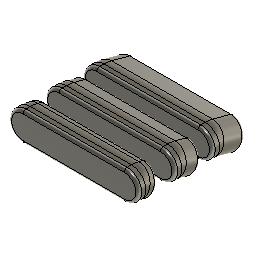
ID.3 Qi charger phone offset (Autodesk Fusion 360 design; units mm, degrees)
part number: 2026-03-30-21-57-16-208
Autodesk Fusion 360 part; units mm, degrees
sketch "Sketch2" plane through (0, 0, 0) normal (0, 1, 0) x (1, 0, 0)
  line L0 (10, 0) -> (80, 0)
  line L1 (80, -20) -> (10, -20)
  arc A0 (0, -10) -> (10, -20) centre (10, -10) ccw
  arc A1 (10, 0) -> (0, -10) centre (10, -10) ccw
  arc A2 (90, -10) -> (80, 0) centre (80, -10) ccw
  arc A3 (80, -20) -> (90, -10) centre (80, -10) ccw
  point P0 (90, 0)
  point P1 (0, -20)
  dimension "d3" = 90
  dimension "d4" = 20
  dimension "d5" = 10
  constraint horizontal L0
  constraint horizontal L1
  constraint coincident P1 L1
  constraint tangent L1 A0
  constraint coincident origin L0
  constraint tangent L0 A1
  constraint equal A0 A1
  constraint coincident A0.start A1.end
  constraint coincident P0 L0
  constraint tangent L0 A2
  constraint equal A0 A2
  constraint tangent L1 A3
  constraint equal A0 A3
  constraint coincident A2.start A3.end
  measures "d3" distance of origin P0
  measures "d4" distance of origin P1
  measures "d5" radius of A0
extrude "Extrude1" add sketch "Sketch2" along normal blind 5 makes body 1
revolve "Revolve1" add 1 faces at (56.6667, 5, 13.3333) angle 15 about axis through (80, 5, 0) along (-1, 0, 0) on bodies 1 bodies 1
extrude "Extrude2" add 1 faces at (56.6667, 8.4509, 12.879) along direction (0, 0.965926, -0.258819) blind 5 on bodies 1 bodies 1
copy_body "CopyPasteBodies1" bodies 1 makes body 2
move_body "Move1" bodies 2 to x (1, 0, 0) y (0, 1, 0) z (0, 0, 1) at (0, 25, 0)
extrude "Extrude3" add 1 faces at (56.6667, 38.2805, 11.5849) along direction (0, 0.965926, -0.258819) blind 5 on bodies 2 bodies 2
copy_body "CopyPasteBodies2" bodies 2 makes body 3
move_body "Move2" bodies 3 to x (1, 0, 0) y (0, 1, 0) z (0, 0, 1) at (0, 26, 0)
extrude "Extrude4" add 1 faces at (56.6667, 69.1102, 10.2908) along direction (0, 0.965926, -0.258819) blind 5 on bodies 3 bodies 3
fillet "Fillet1" radius 2 8 edges at (90, 73.0771, 5.777) (45, 70.4889, -3.8823) (0, 73.0771, 5.777) (45, 75.6653, 15.4362) (0, 51, 10) (45, 51, 0) (90, 51, 10) (45, 51, 20) on bodies 3
fillet "Fillet2" radius 2 16 edges at (0, 0, 10) (45, 0, 0) (90, 0, 10) (45, 0, 20) (45, 9.8296, -1.2941) (0, 12.4178, 8.3652) (45, 15.006, 18.0244) (90, 12.4178, 8.3652) (0, 25, 10) (45, 25, 0) (90, 25, 10) (45, 25, 20) (90, 42.2474, 7.0711) (45, 39.6593, -2.5882) (0, 42.2474, 7.0711) (45, 44.8356, 16.7303) on bodies 1 2
named bodies: "5mm", "10mm", "15mm"
